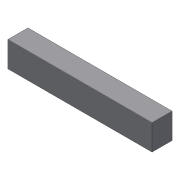
# Autodesk Inventor part: Aluminum Mounting Bridge
Saved by Autodesk Inventor 2015 (Build 190159000, 159)
## iProperties
Created: 2020-01-08
Part Number: Aluminum Mounting Bridge
Material: Generic
Document SubType Name: Modeling
Designer: Ghassan Yusuf
Density: 1 g/cm^3
Appearance: Default
Author: Ghassan Yusuf
Autodesk Inventor part; units mm, degrees
ref_plane "YZ Plane" through (0, 0, 0) normal (1, 0, 0) x (0, 1, 0)
ref_plane "XZ Plane" through (0, 0, 0) normal (0, 1, 0) x (-1, 0, 0)
ref_plane "XY Plane" through (0, 0, 0) normal (0, 0, 1) x (1, 0, 0)
sketch "Sketch1" plane through (0, 0, 0) normal (0, 0, 1) x (1, 0, 0)
  line L0 (-47, 6.4) -> (47, 6.4)
  line L1 (47, 6.4) -> (47, -6.4)
  line L2 (47, -6.4) -> (-47, -6.4)
  line L3 (-47, -6.4) -> (-47, 6.4)
  point P0 (0, 0)
  point P1 (-47, 0)
  point P2 (0, 6.4)
  dimension "d0" = 94
  dimension "d1" = 12.8
  constraints: 8 end point, 2 midpoint, 2 parallel, 1 horizontal, 1 horizontal alignment, 1 perpendicular, 1 vertical alignment
  measures "d0" distance of L0.start L0.end
  measures "d1" distance of L2.end L0.start
extrude "Extrusion1" add sketch "Sketch1" along normal blind 16
chamfer "Chamfer1" distance 0.2 angle 45 12 edges at (0, 6.4, 16) (-47, 0, 16) (-47, 6.4, 8) (0, 6.4, 0) (0, -6.4, 16) (0, -6.4, 0) (47, -6.4, 8) (47, 6.4, 8) (47, 0, 16) (47, 0, 0) (-47, 0, 0) (-47, -6.4, 8)
sketch "Sketch2" plane through (-46.8, 6.4, 0.2) normal (0, 1, 0) x (1, 0, 0)
  circle A0 centre (5.3, -2.8) radius 1.5
  circle A1 centre (5.3, -12.8) radius 1.5
  line L0 (0, -15.8) -> (93.6, -15.8) projected
  line L1 (93.6, 0.2) -> (0, 0.2) projected
  line L2 (-0.2, 0) -> (-0.2, -15.6) projected
  line L3 (7.8, 0.2) -> (7.8, -15.8)
  point P0 (46.8, 0.2)
  dimension "d7" = 3
  dimension "d8" = 10
  dimension "d9" = 16
  dimension "d10" = 3
  dimension "d11" = 5.5
  dimension "d12" = 8
  constraints: 2 centre point, 2 end point, 2 point on line, 1 equal radius, 1 vertical, 1 vertical alignment
  measures "d7" diameter of A0
  measures "d8" distance of A1.centre A0.centre
  measures "d9" distance between parallel lines of L0 L1
  measures "d10" distance from line of L1 A0.centre
  measures "d11" distance from line of L2 A1.centre
  measures "d12" distance between parallel lines of L2 L3
extrude "Extrusion2" cut sketch "Sketch2" against normal blind 5
thread "Thread1" size "M3x0.5" class "6H" standard "ANSI Metric M Profile" full length
thread "Thread2" size "M3x0.5" class "6H" standard "ANSI Metric M Profile" full length
chamfer "Chamfer2" distance 0.2 angle 45 2 edges at (-43, 6.4, 13) (-43, 6.4, 3)
sketch "Sketch3" plane through (-46.8, -6.4, 15.8) normal (0, -1, 0) x (1, 0, 0)
  circle A0 centre (4.8, -7.8) radius 1.6
  circle A1 centre (88.8, -7.8) radius 1.6
  line L0 (0, -15.6) -> (0, 0) projected
  line L1 (93.6, 0) -> (93.6, -15.6) projected
  line L2 (-0.2, 0) -> (-0.2, -15.6) projected
  line L3 (93.8, -15.6) -> (93.8, 0) projected
  point P0 (46.8, -15.8)
  point P1 (0, -7.8)
  point P2 (93.6, -7.8)
  dimension "d22" = 3.2
  dimension "d23" = 5
  dimension "d24" = 5
  constraints: 2 centre point, 2 horizontal alignment, 2 midpoint, 1 equal radius
  measures "d22" diameter of A0
  measures "d23" distance from line of L2 A0.centre
  measures "d24" distance from line of L3 A1.centre
extrude "Extrusion3" cut sketch "Sketch3" against normal blind 5
thread "Thread3" size "M3.5x0.6" class "6H" standard "ANSI Metric M Profile" full length
thread "Thread4" size "M3.5x0.6" class "6H" standard "ANSI Metric M Profile" full length
equation "\"d10\" = -0.5 * d8 + 0.5 * d9"
body "Solid1"
